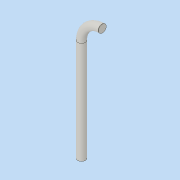
# Autodesk Inventor part: 3mmControlSurfaceShaft_1
Saved by Autodesk Inventor 2017 (Build 210142000, 142)
## iProperties
Created: 2016-10-13
Part Number: 3mmControlSurfaceShaft_1
Material: Generic
Document SubType Name: Modeling
Designer: techn
Density: 1 g/cm^3
Appearance: Steel
Author: techn
Autodesk Inventor part; units mm, degrees
ref_plane "YZ Plane" through (0, 0, 0) normal (1, 0, 0) x (0, 1, 0)
ref_plane "XZ Plane" through (0, 0, 0) normal (0, 1, 0) x (-1, 0, 0)
ref_plane "XY Plane" through (0, 0, 0) normal (0, 0, 1) x (1, 0, 0)
sketch "Sketch1" plane through (0, 0, 0) normal (0, 0, 1) x (1, 0, 0)
  line L0 (0, 0) -> (0, 39.37)
  line L1 (0, 39.37) -> (7.9375, 39.37)
  line L2 (7.9375, 39.37) -> (7.9375, 47.3075)
  line L3 (7.9375, 47.3075) -> (8.0645, 47.3075)
  arc A0 (7.9375, 47.3075) -> (0, 39.37) centre (7.9375, 39.37) ccw
  dimension "d0" = 39.37
  dimension "d1" = 7.9375
  dimension "d2" = 7.9375
  dimension "d3" = 0.127
  constraints: 8 end point, 3 perpendicular, 2 point on circle, 1 centre point, 1 tangent, 1 vertical
  measures "d0" distance of L0.start L0.end
  measures "d1" distance of L0.end L1.end
  measures "d2" distance of L1.end L2.end
  measures "d3" distance of L2.end L3.end
sketch "Sketch2" plane through (0, 0, 0) normal (0, 1, 0) x (-1, 0, 0)
  circle A0 centre (0, 0) radius 1.5
  dimension "d4" = 3
  constraints: 1 centre point, 1 coincident
  measures "d4" diameter of A0
sweep "Sweep1" add profiles "Sketch2" path "Sketch1" path curves L0 A0 L3
body "Solid1"
